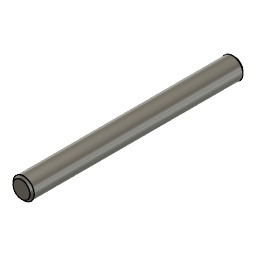
pilar_camara (Autodesk Fusion 360 design; units mm, degrees)
part number: 2026-03-01-15-33-11-237
Autodesk Fusion 360 part; units mm, degrees
sketch "Boceto1" plane through (0, 0, 0) normal (0, 0, 1) x (1, 0, 0)
  circle A0 centre (0, 0) radius 5
  dimension "d1" = 10
  constraint coincident A0.centre origin
  measures "d1" diameter of A0
extrude "Extruir1" add sketch "Boceto1" along normal blind 100
chamfer "Chaflán1" distance 1 angle 45 2 edges at (-4.6616, -1.8081, 100) (-4.6616, -1.8081, 0)
